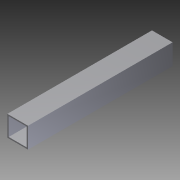
# Autodesk Inventor part: 4 in 1-16 tubing
Saved by Autodesk Inventor 2011 (Build 150239000, 239)
## iProperties
Created: 2013-01-20
Part Number: 4 in 1-16 tubing
Document SubType Name: Modeling
Designer: Danny
Density: 1 g/cm^3
Author: Danny
Autodesk Inventor part; units mm, degrees
ref_plane "YZ Plane" through (0, 0, 0) normal (1, 0, 0) x (0, 1, 0)
ref_plane "XZ Plane" through (0, 0, 0) normal (0, 1, 0) x (-1, 0, 0)
ref_plane "XY Plane" through (0, 0, 0) normal (0, 0, 1) x (1, 0, 0)
sketch "Sketch1" plane through (0, 0, 0) normal (0, 0, 1) x (1, 0, 0)
  line L0 (-25.4, -25.4) -> (0, -25.4)
  line L1 (0, -25.4) -> (0, 0)
  line L2 (0, 0) -> (-25.4, 0)
  line L3 (-25.4, 0) -> (-25.4, -25.4)
  line L4 (-23.8125, -23.8125) -> (-1.5875, -23.8125)
  line L5 (-1.5875, -23.8125) -> (-1.5875, -1.5875)
  line L6 (-1.5875, -1.5875) -> (-23.8125, -1.5875)
  line L7 (-23.8125, -1.5875) -> (-23.8125, -23.8125)
  dimension "d0" = 25.4
  dimension "d1" = 25.4
  dimension "d2" = 22.225
  dimension "d3" = 22.225
  constraints: 16 end point, 4 parallel, 2 horizontal, 2 perpendicular
  measures "d0" distance of L2.end L1.end
  measures "d1" distance of L1.end L0.end
  measures "d2" distance of L6.end L5.end
  measures "d3" distance of L5.end L4.end
extrude "Extrusion1" add sketch "Sketch1" along normal blind 228.6
body "Solid1"
